link lower control (Autodesk Fusion 360 design; units mm, degrees)
Autodesk Fusion 360 part; units mm, degrees
sketch "Sketch1" plane through (0, 0, 28.75) normal (0, 0, -1) x (1, 0, 0)
  circle A0 centre (20, -28.8333) radius 2.95
  circle A1 centre (20, -28.8333) radius 5
  circle A2 centre (20, -68.8333) radius 2.95
  circle A3 centre (20, -68.8333) radius 5
  line L0 (15, -68.8333) -> (25, -68.8333) construction
  line L1 (25, -68.8333) -> (25, -28.8333)
  line L2 (25, -28.8333) -> (15, -28.8333) construction
  line L3 (15, -28.8333) -> (15, -68.8333)
  circle A4 centre (20, -28.8333) radius 2.95
  circle A5 centre (20, -28.8333) radius 2.95
  circle A6 centre (20, -28.8333) radius 3.05
  circle A7 centre (20, -68.8333) radius 3.05
  dimension "d178" = 10
  dimension "d179" = 10
  dimension "d180" = 0.1
  dimension "d181" = 0.1
  dimension "d1" = 40
  constraint concentric A0 A1
  constraint concentric A2 A3
  constraint horizontal L0
  constraint vertical L1
  constraint horizontal L2
  constraint vertical L3
  constraint coincident A1 L1.end
  constraint coincident A3 L0.start
  constraint midpoint A0.centre L2
  constraint concentric A0 A4
  measures "d178" diameter of A1
  measures "d179" diameter of A3
  measures "d1" distance of A0.centre A2.centre
extrude "Extrude1" add sketch "Sketch1" against normal blind 4 contours A1 | A1 A3 L1 L3 | A3
chamfer "Chamfer1" distance 1.5 angle 45 2 edges at (17.1564, 27.7304, 28.75) (17.1564, 69.9363, 32.75)
